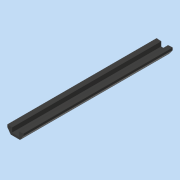
# Autodesk Inventor part: WireGuideToMiniSubExtender
Saved by Autodesk Inventor 2017 (Build 210142000, 142)
## iProperties
Created: 2018-03-28
Part Number: WireGuideToMiniSubExtender
Material: ABS Plastic
Document SubType Name: Modeling
Designer: Derek Wider
Density: 1.06 g/cm^3
Appearance: Smooth - Black
Author: Derek Wider
Autodesk Inventor part; units mm, degrees
ref_plane "YZ Plane" through (0, 0, 0) normal (1, 0, 0) x (0, 1, 0)
ref_plane "XZ Plane" through (0, 0, 0) normal (0, 1, 0) x (-1, 0, 0)
ref_plane "XY Plane" through (0, 0, 0) normal (0, 0, 1) x (1, 0, 0)
sketch "Sketch1" plane through (0, 0, 0) normal (0, 0, 1) x (1, 0, 0)
  line L0 (0, 0) -> (10.795, 0)
  line L1 (10.795, 0) -> (10.795, 4.7625)
  line L2 (0, 0) -> (0, 4.7625)
  arc A0 (0, 4.7625) -> (10.795, 4.7625) centre (5.3975, 55.2749) ccw
  dimension "d0" = 50.8
  dimension "d1" = 10.795
  dimension "d2" = 4.7625
  constraints: 6 end point, 2 point on circle, 1 centre point, 1 horizontal, 1 horizontal alignment, 1 perpendicular, 1 vertical
  measures "d0" radius of A0
  measures "d1" distance of L0.start L0.end
  measures "d2" distance of L0.start L2.end
extrude "Extrusion1" add sketch "Sketch1" along normal blind 101.6
sketch "Sketch2" plane through (0, 0, 101.6) normal (0, 0, 1) x (1, 0, 0)
  arc A0 (0, 4.7625) -> (10.795, 4.7625) centre (5.3975, 55.2749) ccw projected
  line L0 (3.0162, 4.5308) -> (7.7787, 4.5308)
  line L1 (7.7787, 4.5308) -> (7.7787, 1.3558)
  line L2 (7.7787, 1.3558) -> (3.0162, 1.3558)
  line L3 (3.0162, 1.3558) -> (3.0162, 4.5308)
  point P0 (0, 0)
  point P1 (5.3975, 4.5308)
  point P2 (5.3975, 4.4749)
  dimension "d5" = 4.7625
  dimension "d6" = 3.175
  constraints: 8 end point, 3 point on circle, 2 parallel, 1 horizontal, 1 midpoint, 1 perpendicular, 1 vertical alignment
  measures "d5" distance of L1.end L2.end
  measures "d6" distance of L2.end L0.start
extrude "Extrusion2" cut sketch "Sketch2" against normal through all contours A0 L1 L2 L3
chamfer "Chamfer2" distance 3.175 distance2 2.286 1 edges at (0, 0, 50.8) measured on face at (0, 0.5, 50.8)
chamfer "Chamfer3" distance 2.286 distance2 3.175 1 edges at (10.795, 0, 50.8) measured on face at (10.295, 0, 50.8)
body "Solid1"
